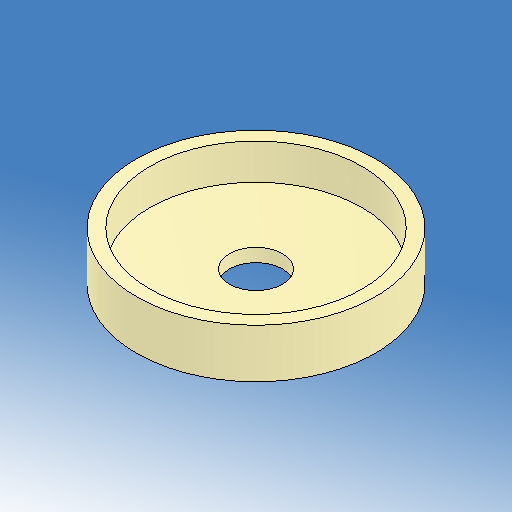
# Autodesk Inventor part: FlipperDriveShaftCap
Saved by Autodesk Inventor 2025 (Build 290162000, 162)
## iProperties
Created: 2024-08-10
Part Number: FlipperDriveShaftCap
Material: Nylon 6/6
Document SubType Name: Modeling
Designer: seene
Density: 1.13 g/cm^3
Appearance: Nylon 6
Author: seene
Autodesk Inventor part; units mm, degrees
ref_plane "YZ Plane" through (0, 0, 0) normal (1, 0, 0) x (0, 1, 0)
ref_plane "XZ Plane" through (0, 0, 0) normal (0, 1, 0) x (-1, 0, 0)
ref_plane "XY Plane" through (0, 0, 0) normal (0, 0, 1) x (1, 0, 0)
sketch "Sketch1" plane through (0, 0, 0) normal (0, 1, 0) x (-1, 0, 0)
  circle A0 centre (0, 0) radius 14.2875
  circle A1 centre (0, 0) radius 3.175
  circle A2 centre (0, 0) radius 12.7
  dimension "d0" = 28.575
  dimension "d1" = 6.35
  dimension "d2" = 1.5875
  constraints: 3 centre point, 2 coincident
  measures "d0" diameter of A0
  measures "d1" diameter of A1
  measures "d2" radial gap between concentric circles of A0 A2
extrude "Extrusion1" add sketch "Sketch1" along normal blind 4.2672 contours A0
extrude "Extrusion2" add sketch "Sketch1" against normal blind 1.5875 contours A0 | A2
body "Solid1"
